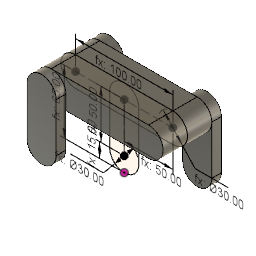
FourLeggedFusionModel.v1 (Autodesk Fusion 360 design; units mm, degrees)
Autodesk Fusion 360 part; units mm, degrees
sketch "Sketch1" plane through (0, 0, 0) normal (0, 1, 0) x (1, 0, 0)
  line L0 (15, -65) -> (15, -15)
  arc A0 (15, -15) -> (-15, -15) centre (0, -15) ccw
  line L1 (-15, -15) -> (-15, -65)
  arc A1 (-15, -65) -> (15, -65) centre (0, -65) ccw
  line L2 (-50, -80) -> (50, -80)
  arc A2 (50, -80) -> (50, -50) centre (50, -65) ccw
  line L3 (50, -50) -> (-50, -50)
  arc A3 (-50, -50) -> (-50, -80) centre (-50, -65) ccw
  line L4 (-50, -65) -> (50, -65) construction
  line L5 (0, -65) -> (0, -15) construction
  dimension "d1" = 30
  dimension "d2" = 50
  dimension "d7" = 30
  dimension "d73" = 15
  dimension "d74" = 65
  dimension "d75" = 50
  dimension "d76" = 100
  measures "d1" diameter of A0
  measures "d2" distance of A1.centre A0.centre
  measures "d7" diameter of A2
  measures "d73" distance of origin A0.centre
  measures "d74" distance of origin A3.centre
  measures "d75" distance of A1.centre A2.centre
  measures "d76" distance of A3.centre A2.centre
extrude "Extrude1" add sketch "Sketch1" along normal mid plane 50 contours L0 L1 A1 L3 | L0 A1 L2 A2 L3 | L1 A1 L2 L3 A3 makes body 1 in component "Torso"
extrude "Extrude1'" add sketch "Sketch1" along normal blind 10 separate body contours L0 L1 A1 L3 | L0 A0 L1 L3 makes body 2 in component "FLLeg"
extrude "Extrude1''" add sketch "Sketch1" against normal blind 10 separate body contours L0 L1 A1 L3 | L0 A0 L1 L3 makes body 3 in component "FRLeg"
extrude "Extrude1'''" add sketch "Sketch1" along normal blind 10 separate body contours L0 L1 A1 L3 | L0 A0 L1 L3 makes body 4 in component "BLLeg"
extrude "Extrude1''''" add sketch "Sketch1" against normal blind 10 separate body contours L0 L1 A1 L3 | L0 A0 L1 L3 makes body 5 in component "BRLeg"
component "Torso" placed x (1, 0, 0) y (0, 1, 0) z (0, 0, 1) at (0, 0, 0)
component "FLLeg" placed x (1, 0, 0) y (0, 1, 0) z (0, 0, 1) at (50, 25, 0)
component "FRLeg" placed x (1, 0, 0) y (0, 1, 0) z (0, 0, 1) at (50, -25, 0)
component "BLLeg" placed x (1, 0, 0) y (0, 1, 0) z (0, 0, 1) at (-50, 25, 0)
component "BRLeg" placed x (1, 0, 0) y (0, 1, 0) z (0, 0, 1) at (-50, -25, 0)
equation "d1 = LegRadius * 2"
equation "d2 = LegLength"
equation "LegRadius = 15.0 mm"
equation "LegLength = 50.0 mm"
equation "BodyLength = 100.0 mm"
equation "BodyWidth = 50 mm"
equation "d7 = LegRadius * 2"
equation "LegWidth = 10.0 mm"
equation "d13 = BodyWidth / 2"
equation "d15 = LegWidth"
equation "d17 = -LegWidth"
equation "d19 = LegWidth"
equation "d21 = -LegWidth"
equation "d73 = LegRadius"
equation "d74 = LegLength + LegRadius"
equation "d75 = BodyLength / 2"
equation "d76 = BodyLength"
